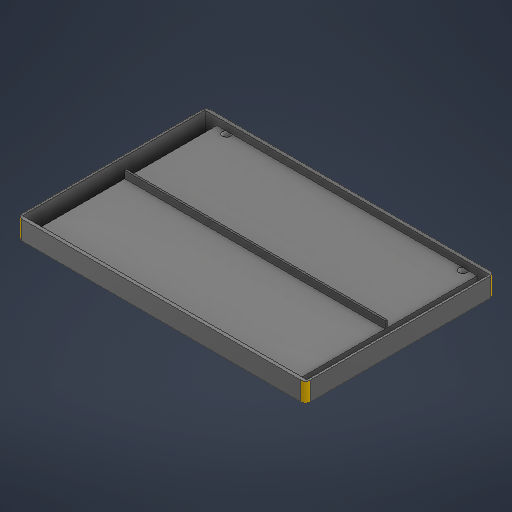
# Autodesk Inventor part: Top_part
Saved by Autodesk Inventor 2027.1 (Build 311270010, 270A)
## iProperties
Created: 2026-09-19
Part Number: Top_part
Material: Ogólny
Document SubType Name: Modeling
Designer: User
Density: 1 g/cm^3
Appearance: Domyślna
Author: User
Autodesk Inventor part; units mm, degrees
ref_plane "YZ Plane" through (0, 0, 0) normal (1, 0, 0) x (0, 1, 0)
ref_plane "XZ Plane" through (0, 0, 0) normal (0, 1, 0) x (-1, 0, 0)
ref_plane "XY Plane" through (0, 0, 0) normal (0, 0, 1) x (1, 0, 0)
sketch "Szkic1" plane through (0, 0, 0) normal (0, 1, 0) x (-1, 0, 0)
  line L0 (-61.8114, 44.3193) -> (58.3886, 44.3193)
  line L1 (58.3886, 44.3193) -> (58.3886, -35.6807)
  line L2 (58.3886, -35.6807) -> (-61.8114, -35.6807)
  line L3 (-61.8114, -35.6807) -> (-61.8114, 44.3193)
  line L4 (-61.8114, 44.3193) -> (58.3886, -35.6807) construction
  line L5 (58.3886, 44.3193) -> (-61.8114, -35.6807) construction
  line L6 (-1.7114, 4.3193) -> (-43.7114, 4.3193)
  line L7 (-1.7114, 4.3193) -> (40.2886, 4.3193) construction
  line L8 (-61.8469, -30.4307) -> (-25.5759, -30.4307)
  line L9 (-25.5759, -30.4307) -> (-25.5759, 39.0693)
  line L10 (-25.5759, 39.0693) -> (-61.8469, 39.0693)
  line L11 (-61.8469, 39.0693) -> (-61.8469, -30.4307)
  line L12 (-61.8469, -30.4307) -> (-25.5759, 39.0693) construction
  line L13 (-25.5759, -30.4307) -> (-61.8469, 39.0693) construction
  line L14 (-1.7114, 4.3193) -> (23.2886, 4.3193)
  line L15 (50.8886, 38.4193) -> (-4.3114, 38.4193)
  line L16 (-4.3114, 38.4193) -> (-4.3114, -29.7807)
  line L17 (-4.3114, -29.7807) -> (50.8886, -29.7807)
  line L18 (50.8886, -29.7807) -> (50.8886, 38.4193)
  line L19 (50.8886, 38.4193) -> (-4.3114, -29.7807) construction
  line L20 (-4.3114, 38.4193) -> (50.8886, -29.7807) construction
  line L21 (-63.7114, -35.6807) -> (60.2886, -35.6807)
  line L22 (60.2886, -35.6807) -> (60.2886, 44.3193)
  line L23 (60.2886, 44.3193) -> (-63.7114, 44.3193)
  line L24 (-63.7114, 44.3193) -> (-63.7114, -35.6807)
  line L25 (-63.7114, -35.6807) -> (60.2886, 44.3193) construction
  line L26 (60.2886, -35.6807) -> (-63.7114, 44.3193) construction
  point P0 (0, 0)
  point P1 (-61.8114, -35.6807)
  dimension "d0" = 120.2
  dimension "d1" = 80
  dimension "d2" = 42
  dimension "d3" = 180
  dimension "d4" = 36.271
  dimension "d5" = 69.5
  dimension "d6" = 25
  dimension "d7" = 55.2
  dimension "d8" = 68.2
  dimension "d9" = 124
  dimension "d10" = 80
  constraints: 54 end point, 8 midpoint, 8 parallel, 6 horizontal, 4 perpendicular, 1 collinear, 1 point on line
  measures "d0" distance of L4.start L1.start
  measures "d1" distance of L1.start L1.end
  measures "d2" distance of L14.start L6.end
  measures "d3" angle of L6 L7
  measures "d4" distance of L10.end L9.end
  measures "d5" distance of L9.end L9.start
  measures "d6" distance of L14.start L14.end
  measures "d7" distance of L18.start L19.end
  measures "d8" distance of L19.end L20.start
  measures "d9" distance of L26.end L22.end
  measures "d10" distance of L22.end L22.start
extrude "Wyciągnięcie proste1" add sketch "Szkic1" along normal blind 5 contours L0 L1 L2 L3 L8 L9 L10 | L3 L10 L11 L8 L21 L24 L23 | L23 L22 L21 L1 | L10 L9 L8 L3 | L3 L8 L11 L10 | L18 L17 L16 L15
move faces "Przesuń1" translate (-3, 0, 0) faces at (63.7114, 1.6667, 17.6527)
sketch "Szkic2" plane through (0, 5, 0) normal (0, 1, 0) x (1, 0, 0)
  line L0 (-60.2886, 35.6807) -> (-60.2886, -44.3193) projected
  line L1 (60.7114, 35.6807) -> (-60.2886, 35.6807) projected
  line L2 (-60.2886, -44.3193) -> (60.7114, -44.3193)
  line L3 (60.7114, -44.3193) -> (60.7114, 35.6807)
  line L4 (60.7114, 35.6807) -> (-60.2886, 35.6807)
  line L5 (-60.2886, 35.6807) -> (-60.2886, -44.3193)
  line L6 (-60.2886, -44.3193) -> (60.7114, 35.6807) construction
  line L7 (60.7114, -44.3193) -> (-60.2886, 35.6807) construction
  line L8 (0.2114, -4.3193) -> (0.2114, -23.8193) construction
  line L9 (0.2114, -4.3193) -> (19.7114, -4.3193) construction
  line L10 (60.3114, -42.9193) -> (-59.8886, -42.9193)
  line L11 (-59.8886, -42.9193) -> (-59.8886, -4.7193)
  line L12 (-59.8886, -4.7193) -> (60.3114, -4.7193)
  line L13 (60.3114, -4.7193) -> (60.3114, -42.9193)
  line L14 (60.3114, -42.9193) -> (-59.8886, -4.7193) construction
  line L15 (-59.8886, -42.9193) -> (60.3114, -4.7193) construction
  line L16 (0.2114, -4.3193) -> (-2.5308, -4.3193)
  line L17 (60.3114, 34.2807) -> (-59.8886, 34.2807)
  line L18 (-59.8886, 34.2807) -> (-59.8886, -3.9193)
  line L19 (-59.8886, -3.9193) -> (60.3114, -3.9193)
  line L20 (60.3114, -3.9193) -> (60.3114, 34.2807)
  line L21 (60.3114, -42.9193) -> (55.3114, -42.9193)
  line L22 (55.3114, -42.9193) -> (55.3114, 34.2807)
  line L23 (55.3114, 34.2807) -> (60.3114, 34.2807)
  line L24 (60.3114, 34.2807) -> (60.3114, -42.9193)
  line L25 (-59.8886, -42.9193) -> (-54.8886, -42.9193)
  line L26 (-54.8886, -42.9193) -> (-54.8886, 34.2807)
  line L27 (-54.8886, 34.2807) -> (-59.8886, 34.2807)
  line L28 (-59.8886, 34.2807) -> (-59.8886, -42.9193)
  point P0 (-59.8886, -4.7193)
  dimension "d26" = 19.5
  dimension "d27" = 90
  dimension "d28" = 120.2
  dimension "d29" = 38.2
  dimension "d30" = 5
  dimension "d31" = 5
  constraints: 54 end point, 8 parallel, 5 horizontal, 5 perpendicular, 4 symmetric about line, 3 midpoint, 3 point on line, 1 vertical
  measures "d26" distance of L8.start L8.end
  measures "d27" angle of L8 L9
  measures "d28" distance of L11.end L12.end
  measures "d29" distance of L10.end L11.end
  measures "d30" distance of L22.end L23.end
  measures "d31" distance of L27.end L26.end
extrude "Wyciągnięcie proste2" add sketch "Szkic2" along normal blind 3 contours L1 L3 L2 L0 | L12 L22 L19 L24 | L12 L26 L19 L22 | L12 L28 L19 L26
extrude "Wyciągnięcie proste3" cut sketch "Szkic2" along normal mid plane 16 contours L10 L22 L12 L13 | L12 L22 L19 L24 | L10 L11 L12 L26 | L19 L22 L17 L20 | L12 L28 L19 L26 | L19 L18 L17 L26
fillet "Zaokrąglenie1" radius 2 4 edges at (60.7114, 4, 44.3193) (60.7114, 4, -35.6807) (-60.2886, 4, -35.6807) (-60.2886, 4, 44.3193)
move faces "Przesuń2" translate (0.5, 0, 0) faces at (60.7114, 5.3333, -8.3473)
move faces "Przesuń3" translate (-0.5, 0, 0) faces at (-60.2886, 5.3333, -8.3473)
sketch "Szkic3" plane through (0, 0, 0) normal (0, -1, 0) x (1, 0, 0)
  arc A0 (61.2114, 42.3193) -> (59.2114, 44.3193) centre (59.2114, 42.3193) ccw
  line L0 (59.2114, 44.3193) -> (-58.7886, 44.3193)
  arc A1 (-58.7886, 44.3193) -> (-60.7886, 42.3193) centre (-58.7886, 42.3193) ccw
  line L1 (-60.7886, 42.3193) -> (-60.7886, -33.6807)
  arc A2 (-60.7886, -33.6807) -> (-58.7886, -35.6807) centre (-58.7886, -33.6807) ccw
  line L2 (-58.7886, -35.6807) -> (59.2114, -35.6807)
  arc A3 (59.2114, -35.6807) -> (61.2114, -33.6807) centre (59.2114, -33.6807) ccw
  line L3 (61.2114, -33.6807) -> (61.2114, 42.3193)
  line L4 (-15.9241, 4.3193) -> (56.5759, 4.3193)
  line L5 (59.2114, -33.6807) -> (-58.7886, 42.3193) construction
  line L6 (-58.7886, -33.6807) -> (59.2114, 42.3193) construction
  line L7 (-60.7886, -35.6807) -> (61.2114, -35.6807)
  line L8 (61.2114, -35.6807) -> (61.2114, 44.3193)
  line L9 (61.2114, 44.3193) -> (-60.7886, 44.3193)
  line L10 (-60.7886, 44.3193) -> (-60.7886, -35.6807)
  line L11 (-60.7886, -35.6807) -> (61.2114, 44.3193) construction
  line L12 (61.2114, -35.6807) -> (-60.7886, 44.3193) construction
  line L13 (0.2114, 4.3193) -> (0.2114, -35.6807) construction
  line L14 (0.2114, 4.3193) -> (61.2114, 4.3193)
  line L15 (0.2114, -35.6807) -> (0.2114, -33.1807) construction
  line L16 (0.2114, -33.1807) -> (50.2114, -33.1807) construction
  circle A4 centre (50.2114, -33.1807) radius 1.5
  circle A5 centre (50.2114, -33.1807) radius 1.75
  circle A6 centre (-49.7886, -33.1807) radius 1.5
  circle A7 centre (-49.7886, -33.1807) radius 1.75
  circle A8 centre (50.2114, 41.8193) radius 1.75
  circle A9 centre (50.2114, 41.8193) radius 1.5
  circle A10 centre (-49.7886, 41.8193) radius 1.5
  circle A11 centre (-49.7886, 41.8193) radius 1.75
  arc A12 (-58.7886, 44.3193) -> (-60.7886, 42.3193) centre (-58.7886, 42.3193) ccw projected
  line L17 (-60.7886, -33.6807) -> (-60.7886, 42.3193) projected
  arc A13 (-60.7886, -33.6807) -> (-58.7886, -35.6807) centre (-58.7886, -33.6807) ccw projected
  line L18 (59.2114, -35.6807) -> (-58.7886, -35.6807) projected
  arc A14 (59.2114, -35.6807) -> (61.2114, -33.6807) centre (59.2114, -33.6807) ccw projected
  line L19 (61.2114, 42.3193) -> (61.2114, -33.6807) projected
  arc A15 (61.2114, 42.3193) -> (59.2114, 44.3193) centre (59.2114, 42.3193) ccw projected
  line L20 (-58.7886, 44.3193) -> (59.2114, 44.3193) projected
  line L21 (-54.8886, 42.9193) -> (-54.8886, -34.2807) projected
  line L22 (-54.8886, -34.2807) -> (-59.8886, -34.2807) projected
  line L23 (-59.8886, -34.2807) -> (-59.8886, 42.9193) projected
  line L24 (-59.8886, 42.9193) -> (-54.8886, 42.9193) projected
  line L25 (55.3114, 42.9193) -> (60.3114, 42.9193) projected
  line L26 (60.3114, 42.9193) -> (60.3114, -34.2807) projected
  line L27 (60.3114, -34.2807) -> (55.3114, -34.2807) projected
  line L28 (55.3114, -34.2807) -> (55.3114, 42.9193) projected
  line L29 (0.2114, 44.3193) -> (0.2114, -35.6807) construction
  line L30 (-60.7886, 4.3193) -> (61.2114, 4.3193) construction
  line L31 (-60.7886, -35.6807) -> (61.2114, -35.6807)
  line L32 (61.2114, -35.6807) -> (61.2114, 44.3193)
  line L33 (61.2114, 44.3193) -> (-60.7886, 44.3193)
  line L34 (-60.7886, 44.3193) -> (-60.7886, -35.6807)
  line L35 (-60.7886, -35.6807) -> (61.2114, 44.3193) construction
  line L36 (61.2114, -35.6807) -> (-60.7886, 44.3193) construction
  point P0 (0, 0)
  point P1 (-1.2886, 4.3193)
  point P2 (0.2114, 4.3193)
  dimension "d41" = 80
  dimension "d42" = 2.5
  dimension "d43" = 50
  dimension "d44" = 90
  dimension "d45" = 3
  dimension "d46" = 3.5
  dimension "d47" = 122
  dimension "d48" = 80
  constraints: 50 end point, 12 centre point, 12 midpoint, 8 point on circle, 6 symmetric about line, 5 coincident, 4 parallel, 3 perpendicular, 2 horizontal, 1 point on line, 6 other
  measures "d41" distance of L8.end L8.start
  measures "d42" distance of L15.start L15.end
  measures "d43" distance of L15.end L16.end
  measures "d44" angle of L15 L16
  measures "d45" diameter of A4
  measures "d46" diameter of A5
  measures "d47" distance of L33.end L32.end
  measures "d48" distance of L32.end L31.end
extrude "Wyciągnięcie proste4" cut sketch "Szkic3" against normal blind 5 contours A4 | A5 | A6 | A7 | A8 | A9 | A10 | A11
